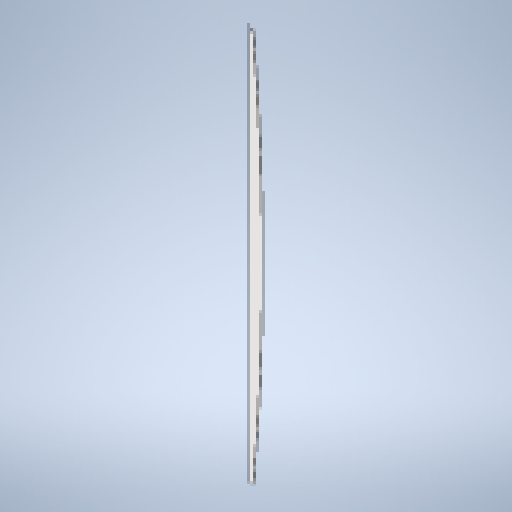
# Autodesk Inventor part: MSC 079 creen pillar
Saved by Autodesk Inventor 2025 (Build 290162010, 162A)
## iProperties
Created: 2024-04-18
Part Number: MSC 079 creen pillar
Material: AISI304
Document SubType Name: Sheet Metal
Designer: admin
Stock Number: МОО 024 лист борт основной
Mass: 48027.3 g
Surface Area: 40202.8 cm^2
Volume: 6003.41 cm^3
Density: 8 g/cm^3
Sheet Metal Rule: AISI304 3mm
Sheet Metal Width: 0,000 mm
Sheet Metal Length: 0,000 mm
Sheet Metal Area: 0,000 mm^2
Appearance: Default
Author: admin
Autodesk Inventor part; units mm, degrees
ref_plane "YZ Plane" through (0, 0, 0) normal (1, 0, 0) x (0, 1, 0)
ref_plane "XZ Plane" through (0, 0, 0) normal (0, 1, 0) x (-1, 0, 0)
ref_plane "XY Plane" through (0, 0, 0) normal (0, 0, 1) x (1, 0, 0)
sketch "Sketch1" plane through (0, 0, 0) normal (0, 0, 1) x (1, 0, 0)
  line L0 (0, 100) -> (0, 50) construction
  line L1 (0, 47) -> (0, 0) construction
  line L2 (0, 50) -> (0, 47) construction
  arc A0 (19.941, -2049.8235) -> (19.2453, 0) centre (-10982.7722, -1028.646) ccw
  line L3 (19.941, -2049.8235) -> (0, -2049.8235)
  line L4 (0, -2049.8235) -> (0, 0)
  line L5 (0, 0) -> (19.2453, 0)
  dimension "d115" = 3
  dimension "d131" = 11050
  dimension "d132" = 19.2453
  dimension "d133" = 19.941
  dimension "d134" = 2049.8235
  measures "d115" distance of L0.end L1.start
  measures "d131" radius of A0
  measures "d132" distance of L1.end L5.end
  measures "d133" distance of L3.start L3.end
  measures "d134" distance of L1.end L3.end
extrude "Plate3" add sketch "Sketch1" along normal blind 3
sketch "Sketch2" plane through (2.1213, -2049.8235, 0.8787) normal (-0.7071068, 0, 0.7071068) x (0, -1, 0)
  line L0 (-2049.8235, 0) -> (0, 0)
  line L1 (0, 0) -> (0, 40)
  line L2 (0, 40) -> (-2049.8235, 40)
  line L3 (-2049.8235, 40) -> (-2049.8235, 0)
  constraints: 6 end point, 1 horizontal, 1 perpendicular, 1 vertical
edge flange "Flange1" height 40 angle 45 thickness 3 bend radius 5 thickness toward (-0.7071068, 0, 0.7071068) relief round relief width 3 relief depth 1.5 edges at (0, -1024.9117, 3) wall of the first edge with corners at (2.1213, 0, 0.8787) (2.1213, -2049.8235, 0.8787) (-26.163, -2049.8235, -27.4056) (-26.163, 0, -27.4056)
bend "Bend3"
corner "Corner3"
equation "\"BendReliefWidth\" = Thickness"
equation "\"BendReliefDepth\" = 0.5 * Thickness"
equation "\"CornerReliefSize\" = 4 * Thickness"
equation "\"MinimumRemnant\" = 2 * Thickness"
equation "\"GapSize\" = Thickness"
equation "\"Thickness\" = 3"
body "Solid4"
